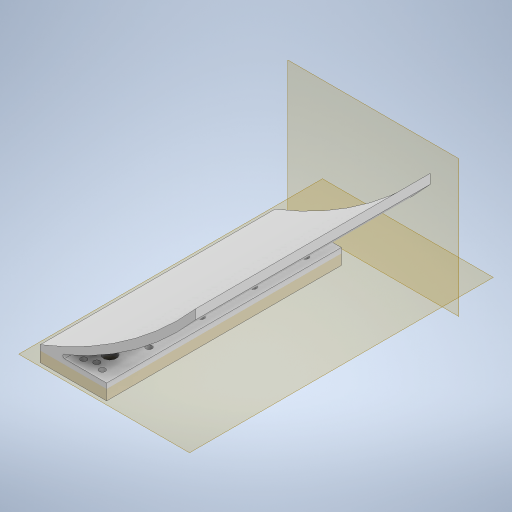
# Autodesk Inventor part: rampside1
Saved by Autodesk Inventor 2023 (Build 270158000, 158)
## iProperties
Created: 2023-10-09
Part Number: rampside1
Material: Generic
Document SubType Name: Modeling
Designer: Avari Mallonee
Density: 1 g/cm^3
Appearance: Default
Author: Avari Mallonee
Autodesk Inventor part; units mm, degrees
ref_plane "YZ Plane" through (0, 0, 0) normal (1, 0, 0) x (0, 1, 0)
ref_plane "XY Plane" through (0, 0, 0) normal (0, 0, 1) x (1, 0, 0)
sketch "Sketch1" plane through (0, 0, 0) normal (0, 1, 0) x (-1, 0, 0)
  point P0 (0, 0)
ref_plane "Work Plane1" through (-14, 16, -288) normal (0, 1, 0) x (1, 0, 0)
sketch "Sketch3" plane through (0, 0, 0) normal (0, 1, 0) x (-1, 0, 0)
  line L0 (14, 0) -> (-14, 0)
  line L1 (14, -144) -> (14, 0)
  line L2 (-14, -144) -> (-14, 0)
  circle A0 centre (5.66, -138.34) radius 1.85
  circle A1 centre (-5.66, -138.34) radius 1.85
  circle A2 centre (0, -136) radius 1.85
  circle A3 centre (-5.66, -74.34) radius 1.85
  circle A4 centre (-5.66, -85.66) radius 1.85
  circle A5 centre (5.66, -85.66) radius 1.85
  circle A6 centre (5.66, -74.34) radius 1.85
  circle A7 centre (8, -80) radius 1.85
  circle A8 centre (-8, -80) radius 1.85
  circle A9 centre (0, -72) radius 1.85
  circle A10 centre (0, -88) radius 1.85
  circle A11 centre (0, -80) radius 4
  circle A12 centre (8, -112) radius 1.85
  circle A13 centre (-8, -112) radius 1.85
  circle A14 centre (0, -104) radius 1.85
  circle A15 centre (0, -120) radius 1.85
  circle A16 centre (0, -112) radius 4
  circle A17 centre (-5.66, -10.34) radius 1.85
  circle A18 centre (-5.66, -21.66) radius 1.85
  circle A19 centre (5.66, -21.66) radius 1.85
  circle A20 centre (5.66, -10.34) radius 1.85
  circle A21 centre (8, -16) radius 1.85
  circle A22 centre (-8, -16) radius 1.85
  circle A23 centre (0, -8) radius 1.85
  circle A24 centre (0, -24) radius 1.85
  circle A25 centre (0, -16) radius 4
  circle A26 centre (8, -48) radius 1.85
  circle A27 centre (-8, -48) radius 1.85
  circle A28 centre (0, -40) radius 1.85
  circle A29 centre (0, -56) radius 1.85
  circle A30 centre (0, -48) radius 4
  circle A31 centre (0, -128) radius 4
  circle A32 centre (0.1754, -96) radius 4
  circle A33 centre (0, -64) radius 4
  circle A34 centre (0, -32) radius 4
  line L3 (14, -144) -> (-14, -144)
  point P0 (0, 0)
  constraints: 35 centre point, 4 end point, 1 perpendicular
extrude "Extrusion1" add sketch "Sketch3" along normal blind 3.175
sketch "Sketch4" plane through (0, 0, 0) normal (0, -1, 0) x (1, 0, 0)
  point P0 (0, 0)
sketch "Sketch10" plane through (-14, 0, 0) normal (0, 0, 1) x (1, 0, 0)
  line L0 (0, 0) -> (28, 0) projected
  line L1 (0, 0) -> (82.55, 0)
  line L2 (82.55, 0) -> (82.55, 69.85)
  line L3 (0, 3.175) -> (28, 3.175) projected
  line L4 (28, 0) -> (28, 3.175) projected
  line L5 (0, 0) -> (0, 3.175) projected
  line L6 (0, 0) -> (-12.7, 0)
  line L7 (-12.7, 3.175) -> (0, 3.175)
  line L8 (0, 3.175) -> (0, 0)
  arc A0 (-3.0407, 3.175) -> (82.55, 64.0105) centre (-82.4635, 205.5441) ccw
  arc A1 (-12.7, 3.175) -> (82.55, 69.85) centre (-103.2617, 233.9221) ccw
  line L9 (-12.7, 3.175) -> (-12.7, 0)
  point P0 (14, 0)
  dimension "d18" = 82.55
  dimension "d19" = 69.85
  constraints: 12 end point, 4 point on circle, 2 centre point, 2 point on line, 1 collinear, 1 horizontal, 1 parallel, 1 vertical
  measures "d18" distance of L0.start L1.end
  measures "d19" distance of L1.end L2.end
extrude "Extrusion7" add sketch "Sketch10" against normal up to surface (144 mm away) contours L6 L9 L7 L5 | L7 A1 L2 A0
fillet "Fillet3" radius 1.016 1 edges at (-17.0407, 3.175, -72)
sketch "Sketch11" plane through (0, 0, 0) normal (0, -1, 0) x (1, 0, 0)
  line L0 (-26.7, 0) -> (14, 0) projected
  line L1 (-26.7, 0) -> (-26.7, -144) projected
  line L2 (14, -144) -> (-26.7, -144) projected
  line L3 (14, 0) -> (14, -144) projected
  circle A0 centre (0, -32) radius 4 projected
  circle A1 centre (-0.1754, -96) radius 4 projected
  circle A2 centre (0, -48) radius 4 projected
  circle A3 centre (0, -40) radius 1.85 projected
  circle A4 centre (-8, -48) radius 1.85 projected
  circle A5 centre (0, -8) radius 1.85 projected
  circle A6 centre (-8, -16) radius 1.85 projected
  circle A7 centre (0, -120) radius 1.85 projected
  circle A8 centre (8, -112) radius 1.85 projected
  circle A9 centre (-5.66, -138.34) radius 1.85 projected
  circle A10 centre (5.66, -138.34) radius 1.85 projected
  circle A11 centre (0, -136) radius 1.85 projected
  circle A12 centre (-8, -80) radius 1.85 projected
  circle A13 centre (8, -80) radius 1.85 projected
  circle A14 centre (0, -72) radius 1.85 projected
  circle A15 centre (0, -88) radius 1.85 projected
  circle A16 centre (-8, -112) radius 1.85 projected
  circle A17 centre (0, -104) radius 1.85 projected
  circle A18 centre (0, -112) radius 4 projected
  circle A19 centre (8, -16) radius 1.85 projected
  circle A20 centre (0, -24) radius 1.85 projected
  circle A21 centre (8, -48) radius 1.85 projected
  circle A22 centre (0, -56) radius 1.85 projected
  circle A23 centre (0, -128) radius 4 projected
  circle A24 centre (0, -64) radius 4 projected
  circle A25 centre (0, -16) radius 4 projected
  circle A26 centre (-5.66, -10.34) radius 1.85 projected
  circle A27 centre (-5.66, -21.66) radius 1.85 projected
  circle A28 centre (5.66, -21.66) radius 1.85 projected
  circle A29 centre (5.66, -10.34) radius 1.85 projected
  circle A30 centre (0, -80) radius 4 projected
  circle A31 centre (-5.66, -74.34) radius 1.85 projected
  circle A32 centre (-5.66, -85.66) radius 1.85 projected
  circle A33 centre (5.66, -85.66) radius 1.85 projected
  circle A34 centre (5.66, -74.34) radius 1.85 projected
  point P0 (0, 0)
extrude "Extrusion8" add sketch "Sketch11" along normal blind 6.35
ref_plane "Work Plane2" through (68.55, 64.0105, 12.7) normal (0, 0, 1) x (1, 0, 0)
mirror "Mirror1" about plane through (68.55, 64.0105, 12.7) normal (0, 0, 1) of "Extrusion1", "Extrusion7", "Fillet3", "Extrusion8"
sketch "Sketch13" plane through (0, -6.35, 0) normal (0, -1, 0) x (1, 0, 0)
  line L0 (-71.1109, -172.9403) -> (93.8528, -172.9403)
  line L1 (93.8528, -172.9403) -> (93.8528, 6.9583)
  line L2 (93.8528, 6.9583) -> (-71.1109, 6.9583)
  line L3 (-71.1109, 6.9583) -> (-71.1109, -172.9403)
  point P0 (0, 0)
  constraints: 8 end point, 2 parallel, 1 horizontal, 1 perpendicular
extrude "Extrusion10" cut sketch "Sketch13" against normal blind 381
body "Solid2"
